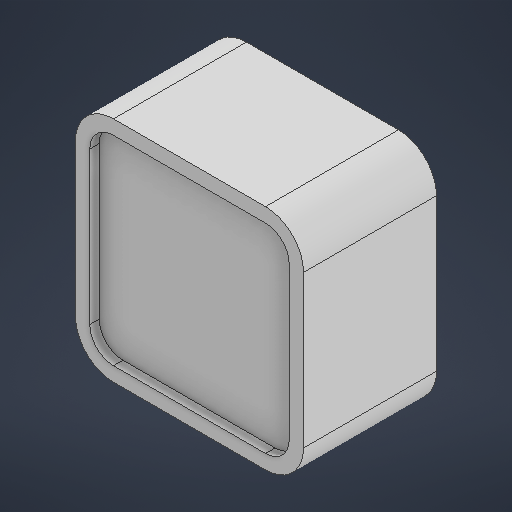
# Autodesk Inventor part: M5Atom
Saved by Autodesk Inventor 2026 (Build 300175050, 175E)
## iProperties
Created: 2026-07-07
Part Number: M5Atom
Material: 一般
Document SubType Name: Modeling
Designer: hanaj
Density: 1 g/cm^3
Appearance: 既定
Author: hanaj
Autodesk Inventor part; units mm, degrees
ref_plane "YZ Plane" through (0, 0, 0) normal (1, 0, 0) x (0, 1, 0)
ref_plane "XZ Plane" through (0, 0, 0) normal (0, 1, 0) x (-1, 0, 0)
ref_plane "XY Plane" through (0, 0, 0) normal (0, 0, 1) x (1, 0, 0)
sketch "スケッチ1" plane through (0, 0, 0) normal (0, 0, 1) x (1, 0, 0)
  line L0 (-12, 12) -> (12, 12)
  line L1 (12, 12) -> (12, -12)
  line L2 (12, -12) -> (-12, -12)
  line L3 (-12, -12) -> (-12, 12)
  line L4 (-12, 12) -> (12, -12) construction
  line L5 (12, 12) -> (-12, -12) construction
  point P0 (0, 0)
  dimension "d0" = 24
  dimension "d1" = 24
  constraints: 12 end point, 2 midpoint, 2 parallel, 1 horizontal, 1 perpendicular
  measures "d0" distance of L1.end L2.end
  measures "d1" distance of L0.end L1.end
extrude "押し出し1" add sketch "スケッチ1" along normal blind 14
fillet "フィレット1" radius 4 4 edges at (-12, 12, 7) (12, 12, 7) (12, -12, 7) (-12, -12, 7)
sketch "スケッチ2" plane through (0, 0, 14) normal (0, 0, 1) x (1, 0, 0)
  arc A0 (-12, -8) -> (-8, -12) centre (-8, -8) ccw projected
  line L0 (-8, -12) -> (8, -12) projected
  arc A1 (8, -12) -> (12, -8) centre (8, -8) ccw projected
  line L1 (12, -8) -> (12, 8) projected
  arc A2 (12, 8) -> (8, 12) centre (8, 8) ccw projected
  line L2 (8, 12) -> (-8, 12) projected
  arc A3 (-8, 12) -> (-12, 8) centre (-8, 8) ccw projected
  line L3 (-12, 8) -> (-12, -8) projected
  line L4 (-8, 10.5) -> (8, 10.5)
  arc A4 (10.5, 8) -> (8, 10.5) centre (8, 8) ccw
  line L5 (10.5, 8) -> (10.5, -8)
  arc A5 (8, -10.5) -> (10.5, -8) centre (8, -8) ccw
  line L6 (8, -10.5) -> (-8, -10.5)
  arc A6 (-10.5, -8) -> (-8, -10.5) centre (-8, -8) ccw
  line L7 (-10.5, -8) -> (-10.5, 8)
  arc A7 (-8, 10.5) -> (-10.5, 8) centre (-8, 8) ccw
  point P0 (0, 0)
  dimension "d5" = 1.5
  constraints: 8 end point, 8 point on circle, 4 centre point, 7 other
  measures "d5" distance between parallel lines of L2 L4
extrude "押し出し2" cut sketch "スケッチ2" against normal blind 1 contours L4 A4 L5 A5 L6 A6 L7 A7
